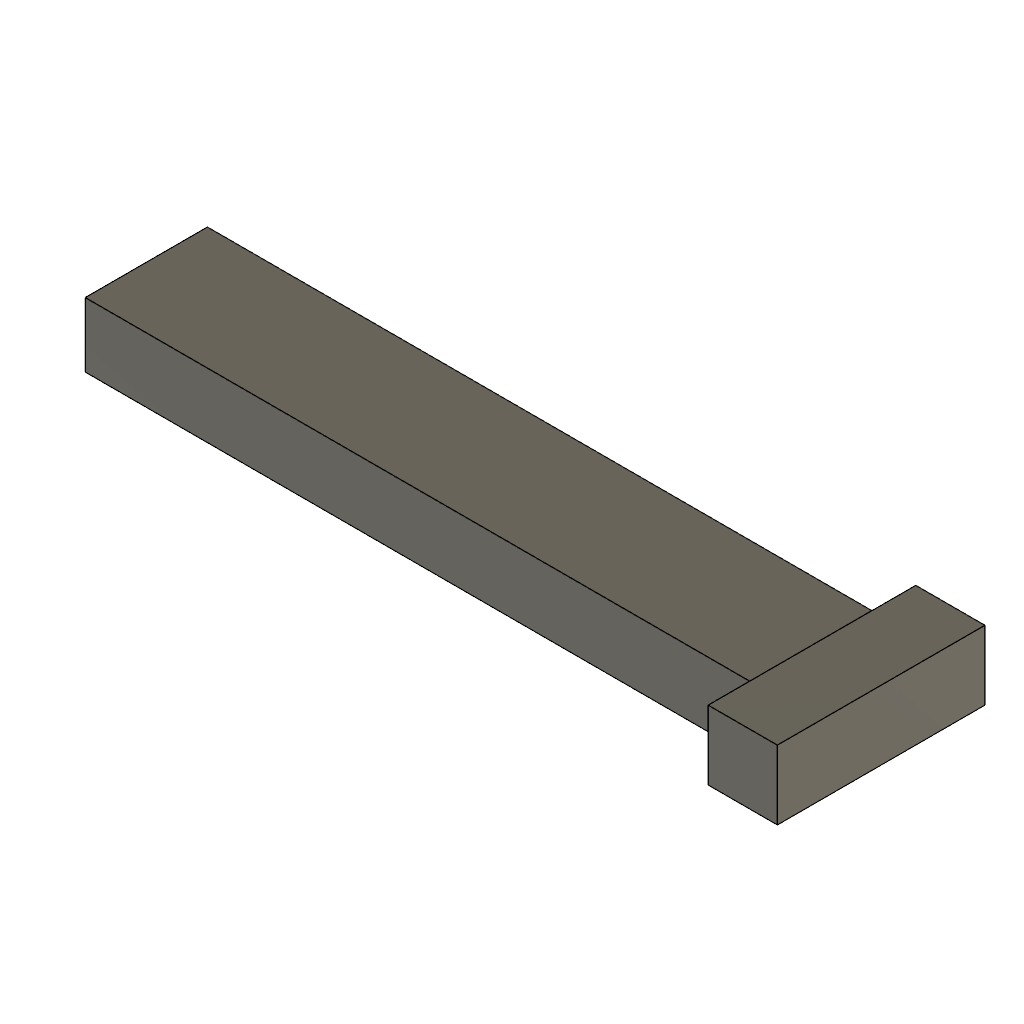
seminaire_FISA-A3_bloque_seringue_20260818 (Autodesk Fusion 360 design; units mm, degrees)
part number: 2026-08-18-10-33-07-482
Autodesk Fusion 360 part; units mm, degrees
sketch "Esquisse1" plane through (0, 0, 0) normal (0, 0, 1) x (1, 0, 0)
  line L0 (0, 0) -> (-29, 0)
  line L1 (-29, 0) -> (-29, 5.3)
  line L2 (-29, 5.3) -> (0, 5.3)
  line L3 (0, 5.3) -> (0, 0)
  dimension "d1" = 5.3
  dimension "d2" = 29
  constraint horizontal L0
  constraint vertical L1
  constraint horizontal L2
  constraint vertical L3
  constraint coincident L0.start L3.end
  measures "d1" distance of L0.end L1.end
  measures "d2" distance of L0.start L0.end
extrude "Extrusion2" add sketch "Esquisse1" along normal blind 2.8
sketch "Esquisse2" plane through (0, 0, 0) normal (0, 0, 1) x (1, 0, 0)
  line L0 (0, 7) -> (3, 7)
  line L1 (3, 7) -> (3, -2)
  line L2 (3, -2) -> (0, -2)
  line L3 (0, -2) -> (0, 7)
  dimension "d7" = 3
  dimension "d8" = 9
  constraint horizontal L0
  constraint vertical L1
  constraint horizontal L2
  constraint vertical L3
  measures "d7" distance of L0.start L0.end
  measures "d8" distance of L0.end L1.end
extrude "Extrusion3" add sketch "Esquisse2" along normal blind 3
